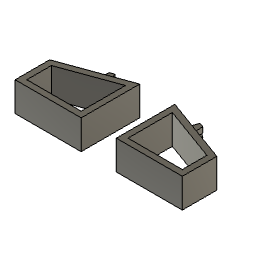
Microfreak Parametric v15 (Autodesk Fusion 360 design; units mm, degrees)
Autodesk Fusion 360 part; units mm, degrees
sketch "Sketch1" plane through (0, 0, 0) normal (0, 0, 1) x (1, 0, 0)
  line L0 (0, 0) -> (112.7631, 0)
  line L1 (112.7631, 0) -> (112.7631, 100)
  line L2 (112.7631, 100) -> (0, 58.9576)
  line L3 (0, 0) -> (0, 58.9576)
  line L4 (10, 10) -> (10, 51.9555)
  line L5 (102.7631, 85.7185) -> (10, 51.9555)
  line L6 (102.7631, 10) -> (102.7631, 85.7185)
  line L7 (10, 10) -> (102.7631, 10)
  dimension "d12" = 100
  dimension "d13" = 70
  dimension "d15" = 120
  constraint coincident L0.start L3.start
  constraint horizontal L0
  constraint perpendicular L0 L1
  constraint perpendicular L0 L3
  measures "d12" distance of L0.end L1.end
  measures "d13" angle of L1 L2
  measures "d15" distance of L1.end L2.end
extrude "Extrude1" add sketch "Sketch1" along normal blind 50 makes body 1
ref_plane "WorkPlane1" through (56.3816, 50, 25) normal (0, 0, -1) x (-1, 0, 0)
sketch "Sketch2" plane through (65.7785, 47.5, 25) normal (0, 0, -1) x (1, 0, 0)
  line L0 (-3.6636, -34.0656) -> (9.4921, -38.8538)
  line L1 (9.4921, -38.8538) -> (4.3618, -52.9492)
  line L2 (4.3618, -52.9492) -> (-3.1557, -50.2131)
  line L3 (-3.1557, -50.2131) -> (-3.6636, -34.0656)
  dimension "d19" = 14
  dimension "d20" = 15
  dimension "d21" = 8
  constraint perpendicular L1 L2
  measures "d19" distance of L0.start L0.end
  measures "d20" distance of L0.end L1.end
  measures "d21" distance of L1.end L2.end
extrude "Extrude2" add sketch "Sketch2" along normal blind 17 from surface at 1 bodies 1
mirror "Mirror1" about plane through (56.3816, 50, 25) normal (0, 0, -1) of "Extrude2"
ref_plane "WorkPlane6" through (62.1149, 81.5656, 26) normal (0.34202, -0.939693, 0) x (0.939693, 0.34202, 0)
sketch "Sketch5" plane through (62.1149, 81.5656, 26) normal (0.34202, -0.939693, 0) x (0.939693, 0.34202, 0)
  line L0 (0, 0) -> (0, 5) construction
  circle A0 through (2.8191, 5, 1.0261) (-1.4095, 7.5981, -0.513) (-1.4095, 2.4019, -0.513)
  dimension "d43" = 6
  constraint coincident L0.start origin
extrude "Extrude5" cut sketch "Sketch5" against normal blind 22.5 contours A0 in plane through (62.1149, 81.5656, 26) normal (0, -1, 0) bodies 1
ref_plane "WorkPlane7" through (142.7631, 50, 25) normal (1, 0, 0) x (0, 1, 0)
mirror "Mirror3" about plane through (142.7631, 50, 25) normal (1, 0, 0) of bodies 1 makes body 2
extrude "Extrude4" [rolled back] along distance 15 taper angle 0
extrude "Extrude3" [rolled back] along distance 22.5 taper angle 0
ref_plane "WorkPlane4" through (142.7631, 50, 25) normal (1, 0, 0) x (0, 1, 0)
mirror "Mirror2" [rolled back] mirror stitch tolerance 0.1
equation "tabHeight = 15 mm" comment "Should not edit this parameter"
equation "tabTopLength = 8 mm" comment "Should not edit this parameter"
equation "tabBottomLength = 14 mm" comment "Should not edit this parameter"
equation "tabSpacer = 2 mm" comment "Should not edit this parameter"
equation "tabCircleRadius = 3 mm" comment "Should not edit this parameter"
equation "tabCircleSpacer = 5 mm" comment "Should not edit this parameter"
equation "tilt = 20 deg" comment "Device tilt"
equation "baseWidth = 50 mm" comment "Stand width"
equation "baseHeight = 100 mm" comment "Stand height"
equation "thickness = 10 mm" comment "Stand thickness"
equation "roundness = 1 mm" comment "Stand roundness"
equation "d12 = baseHeight"
equation "d13 = 90 deg - tilt"
equation "baseLength = 120 mm" comment "Stand length"
equation "d15 = baseLength"
equation "d16 = -thickness"
equation "d17 = baseWidth"
equation "d19 = tabBottomLength"
equation "d20 = tabHeight"
equation "d21 = tabTopLength"
equation "tabWidth = 17 mm" comment "Should not edit this parameter"
equation "d23 = tabSpacer / 2"
equation "d24 = tabWidth"
equation "d32 = tabHeight * 1.5"
equation "d35 = tabHeight"
equation "d37 = tabHeight * 2"
equation "d43 = tabCircleRadius * 2"
equation "d44 = -tabHeight * 1.5"
equation "d46 = 2 * tabHeight"
